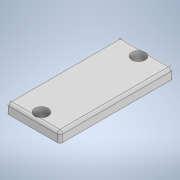
# Autodesk Inventor part: Part2
Saved by Autodesk Inventor 2020.2 (Build 242310000, 310)
## iProperties
Created: 2020-03-08
Part Number: Part2
Material: Generic
Document SubType Name: Modeling
Designer: AOFUser
Density: 1 g/cm^3
Appearance: Default
Author: AOFUser
Autodesk Inventor part; units mm, degrees
ref_plane "YZ Plane" through (0, 0, 0) normal (1, 0, 0) x (0, 1, 0)
ref_plane "XZ Plane" through (0, 0, 0) normal (0, 1, 0) x (-1, 0, 0)
ref_plane "XY Plane" through (0, 0, 0) normal (0, 0, 1) x (1, 0, 0)
sketch "Sketch1" plane through (0, 0, 0) normal (0, 1, 0) x (-1, 0, 0)
  line L0 (0, 0) -> (-16, 0)
  line L1 (-16, 0) -> (-16, -34)
  line L2 (-16, -34) -> (0, -34)
  line L3 (0, -34) -> (0, 0)
  dimension "d0" = 16
  dimension "d1" = 34
  constraints: 8 end point, 2 parallel, 1 horizontal, 1 perpendicular
  measures "d0" distance of L2.end L1.end
  measures "d1" distance of L1.end L0.end
extrude "Extrusion1" add sketch "Sketch1" along normal blind 3
sketch "Sketch2" plane through (0, 3, 0) normal (0, 1, 0) x (1, 0, 0)
  line L0 (0, 0) -> (16, 0) projected
  line L1 (8, 0) -> (8, 2.5)
  line L2 (16, 34) -> (0, 34) projected
  line L3 (8, 34) -> (8, 31.5)
  dimension "d4" = 2.5
  dimension "d5" = 2.5
  constraints: 4 end point, 2 midpoint, 2 vertical
  measures "d4" distance of L1.start L1.end
  measures "d5" distance of L3.start L3.end
hole "Hole1" at (8, 3, -31.5) at (8, 3, -2.5) direction (0, -1, 0) diameter 4 depth 10 tip angle 118
fillet "Fillet1" radius 0.8 8 edges at (0, 1.5, 0) (0, 1.5, -34) (16, 1.5, 0) (16, 1.5, -34) (16, 3, -17) (8, 3, -34) (0, 3, -17) (8, 3, 0)
body "Solid1"
